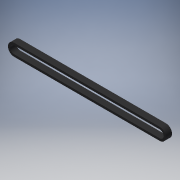
# Autodesk Inventor part: HTD 5M 775
Saved by Autodesk Inventor 2019.4 (Build 234330000, 330)
## iProperties
Created: 2020-01-19
Part Number: HTD 5M 775
Material: Rubber
Document SubType Name: Modeling
Designer: Mark
Mass: 56.8664 g
Surface Area: 314.026 cm^2
Volume: 61.1467 cm^3
Density: 0.93 g/cm^3
Appearance: Rubber - Black
Author: Mark
Autodesk Inventor part; units mm, degrees
ref_plane "YZ Plane" through (0, 0, 0) normal (1, 0, 0) x (0, 1, 0)
ref_plane "XZ Plane" through (0, 0, 0) normal (0, 1, 0) x (-1, 0, 0)
ref_plane "XY Plane" through (0, 0, 0) normal (0, 0, 1) x (1, 0, 0)
sketch "Sketch1" plane through (0, 0, 0) normal (0, 0, 1) x (1, 0, 0)
  arc A0 (0, 11.935) -> (0, -11.935) centre (0, 0) ccw
  arc A1 (350, -11.935) -> (350, 11.935) centre (350, 0) ccw
  line L0 (0, 11.935) -> (350, 11.935)
  line L1 (0, -11.935) -> (350, -11.935)
  line L2 (350, 0) -> (0, 0)
  line L3 (350, 9.305) -> (0, 9.305)
  arc A2 (0, 9.305) -> (0, -9.305) centre (0, 0) ccw
  line L4 (0, -9.305) -> (350, -9.305)
  arc A3 (350, -9.305) -> (350, 9.305) centre (350, 0) ccw
  line L5 (350, 14.565) -> (0, 14.565)
  arc A4 (0, 14.565) -> (0, -14.565) centre (0, 0) ccw
  line L6 (0, -14.565) -> (350, -14.565)
  arc A5 (350, -14.565) -> (350, 14.565) centre (350, 0) ccw
  dimension "d0" = 23.87
  dimension "d1" = 23.87
  dimension "d2" = 350
  dimension "d3" = 350
  dimension "d4" = 2.63
  dimension "d5" = 2.63
  constraints: 14 end point, 12 point on circle, 6 centre point, 4 tangent, 1 coincident, 6 other
  measures "d0" diameter of A0
  measures "d1" diameter of A1
  measures "d2" distance of L2.end L2.start
  measures "d3" distance of L2.start L2.end
  measures "d4" distance between parallel lines of L0 L3
  measures "d5" distance between parallel lines of L0 L5
extrude "Extrusion1" add sketch "Sketch1" along normal blind 15 contours L0 A1 L1 A0 | A5 L6 A4 L5
body "Solid1"
